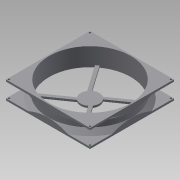
# Autodesk Inventor part: fan_body
Saved by Autodesk Inventor 2015 (Build 190159000, 159)
## iProperties
Created: 2015-05-21
Part Number: fan_body
Material: Generic
Document SubType Name: Modeling
Designer: Joe Sheldon
Density: 1 g/cm^3
Appearance: Default
Author: Joe Sheldon
Autodesk Inventor part; units mm, degrees
ref_plane "YZ Plane" through (0, 0, 0) normal (1, 0, 0) x (0, 1, 0)
ref_plane "XZ Plane" through (0, 0, 0) normal (0, 1, 0) x (-1, 0, 0)
ref_plane "XY Plane" through (0, 0, 0) normal (0, 0, 1) x (1, 0, 0)
sketch "Sketch1" plane through (0, 0, 0) normal (0, 1, 0) x (-1, 0, 0)
  line L0 (0, 0) -> (88.9, 0)
  line L1 (88.9, 0) -> (88.9, -88.9)
  line L2 (88.9, -88.9) -> (0, -88.9)
  line L3 (0, -88.9) -> (0, 0)
  circle A0 centre (44.45, -44.45) radius 43.18
  dimension "d0" = 88.9
  dimension "d1" = 88.9
  dimension "d2" = 86.36
  constraints: 8 end point, 2 parallel, 1 centre point, 1 horizontal, 1 perpendicular
  measures "d0" distance of L1.end L2.end
  measures "d1" distance of L0.end L1.end
  measures "d2" diameter of A0
extrude "Extrusion1" add sketch "Sketch1" along normal blind 23.114
sketch "Sketch2" plane through (0, 23.114, 0) normal (0, 1, 0) x (1, 0, 0)
  line L0 (0, 0) -> (-1.6002, 0)
  line L1 (-1.6002, 0) -> (-1.6002, 1.6002)
  line L2 (-1.6002, 1.6002) -> (0, 1.6002)
  line L3 (0, 1.6002) -> (0, 0)
  line L4 (-88.9, 0) -> (-87.2998, 0)
  line L5 (-87.2998, 0) -> (-87.2998, 1.6002)
  line L6 (-87.2998, 1.6002) -> (-88.9, 1.6002)
  line L7 (-88.9, 1.6002) -> (-88.9, 0)
  line L8 (-88.9, 88.9) -> (-87.2998, 88.9)
  line L9 (-87.2998, 88.9) -> (-87.2998, 87.2998)
  line L10 (-87.2998, 87.2998) -> (-88.9, 87.2998)
  line L11 (-88.9, 87.2998) -> (-88.9, 88.9)
  line L12 (0, 88.9) -> (-1.6002, 88.9)
  line L13 (-1.6002, 88.9) -> (-1.6002, 87.2998)
  line L14 (-1.6002, 87.2998) -> (0, 87.2998)
  line L15 (0, 87.2998) -> (0, 88.9)
  circle A0 centre (-87.2998, 1.6002) radius 0.9525
  circle A1 centre (-87.2998, 87.2998) radius 0.9525
  circle A2 centre (-1.6002, 87.2998) radius 0.9525
  circle A3 centre (-1.6002, 1.6002) radius 0.9525
  dimension "d5" = 1.6002
  dimension "d6" = 1.6002
  dimension "d7" = 1.6002
  dimension "d8" = 1.6002
  dimension "d9" = 1.6002
  dimension "d10" = 1.6002
  dimension "d11" = 1.6002
  dimension "d12" = 1.6002
  dimension "d13" = 1.905
  dimension "d14" = 1.905
  dimension "d15" = 1.905
  dimension "d16" = 1.905
  constraints: 32 end point, 8 parallel, 4 centre point, 4 coincident, 4 horizontal, 4 perpendicular
  measures "d5" distance of L1.end L2.end
  measures "d6" distance of L0.end L1.end
  measures "d7" distance of L6.end L5.end
  measures "d8" distance of L5.end L4.end
  measures "d9" distance of L9.end L10.end
  measures "d10" distance of L8.end L9.end
  measures "d11" distance of L14.end L13.end
  measures "d12" distance of L13.end L12.end
  measures "d13" diameter of A0
  measures "d14" diameter of A1
  measures "d15" diameter of A2
  measures "d16" diameter of A3
extrude "Extrusion2" cut sketch "Sketch2" against normal blind 29.464 contours A3 L2 L1 | L1 L2 A3 | A0 L6 L5 | L5 L6 A0 | A1 L10 L9 | L9 L10 A1 | A2 L14 L13 | L13 L14 A2
sketch "Sketch3" plane through (-88.9, 0, 0) normal (0, 0, 1) x (1, 0, 0)
  line L0 (88.9, 0) -> (0, 0) projected
  line L1 (88.9, 0) -> (88.9, 23.114) projected
  line L2 (0, 23.114) -> (88.9, 23.114) projected
  line L3 (0, 0) -> (0, 23.114) projected
  line L4 (88.9, 0) -> (88.9, 23.114) projected
  line L5 (0, 23.114) -> (88.9, 23.114)
  line L6 (88.9, 23.114) -> (88.9, 21.082)
  line L7 (88.9, 21.082) -> (0, 21.082)
  line L8 (0, 21.082) -> (0, 23.114)
  dimension "d19" = 2.032
  constraints: 8 end point, 2 parallel, 1 horizontal, 1 perpendicular, 1 point on line
  measures "d19" distance of L5.end L6.end
extrude "Extrusion3" cut sketch "Sketch3" against normal blind 96.139 contours L0 L3 L7 L1
sketch "Sketch4" plane through (0, 23.114, 0) normal (0, 1, 0) x (1, 0, 0)
  circle A0 centre (-1.6002, 1.6002) radius 0.9525 projected
  circle A1 centre (-87.2998, 87.2998) radius 0.9525 projected
  circle A2 centre (-87.2998, 1.6002) radius 0.9525 projected
  circle A3 centre (-1.6002, 87.2998) radius 0.9525 projected
  circle A4 centre (-44.45, 44.45) radius 43.18 projected
  line L0 (-88.9, 0) -> (0, 0) projected
  line L1 (0, 0) -> (0, 88.9) projected
  line L2 (0, 88.9) -> (-88.9, 88.9) projected
  line L3 (-88.9, 88.9) -> (-88.9, 0) projected
  circle A5 centre (-44.45, 44.45) radius 44.348
  constraints: 1 centre point
extrude "Extrusion4" add sketch "Sketch4" along normal blind 7.62 contours A5
chamfer "Chamfer1" distance 4.7625 angle 45 1 edges at (-88.798, 23.114, -44.45)
mirror "Mirror1" about plane through (-44.45, 30.734, -44.45) normal (0, 1, 0) of "Extrusion1", "Extrusion4", "Chamfer1", "Extrusion2"
sketch "Sketch5" plane through (-88.9, 61.468, 0) normal (0, 0, 1) x (1, 0, 0)
  line L0 (88.9, 0) -> (0, 0) projected
  line L1 (0, 0) -> (0, -23.114) projected
  line L2 (0, -23.114) -> (23.5685, -23.114) projected
  line L3 (65.3315, -23.114) -> (88.9, -23.114) projected
  line L4 (88.9, 0) -> (88.9, -23.114) projected
  line L5 (88.9, 0) -> (88.9, -23.114) projected
  line L6 (0, -23.114) -> (88.9, -23.114)
  line L7 (88.9, -23.114) -> (88.9, -21.082)
  line L8 (88.9, -21.082) -> (0, -21.082)
  line L9 (0, -21.082) -> (0, -23.114)
  point P0 (88.9, -61.468)
  dimension "d27" = 2.032
  constraints: 8 end point, 2 parallel, 1 horizontal, 1 horizontal alignment, 1 perpendicular, 1 point on line
  measures "d27" distance of L7.end L6.end
extrude "Extrusion5" cut sketch "Sketch5" against normal blind 106.045 contours L4 L8 L1 L0
sketch "Sketch7" plane through (-88.9, 21.082, 0) normal (0, -1, 0) x (1, 0, 0)
  line L0 (75.9799, 0) -> (78.7808, -1.9598)
  line L1 (78.7808, -1.9598) -> (49.7901, -43.3923)
  line L2 (49.7901, -43.3923) -> (46.9892, -41.4325)
  line L3 (46.9892, -41.4325) -> (75.9799, 0)
  point P0 (88.9, 0)
  constraints: 8 end point, 2 parallel, 1 perpendicular
extrude "Extrusion6" add sketch "Sketch7" against normal blind 2.032
pattern_circular "Circular Pattern1" count 4 over 360 about axis through (-44.45, 61.468, -44.45) along (0, 1, 0) of "Extrusion6"
sketch "Sketch8" plane through (-88.9, 21.082, 0) normal (0, -1, 0) x (1, 0, 0)
  arc A0 (23.5685, 0) -> (0, -23.5685) centre (44.45, -44.45) ccw projected
  circle A1 centre (44.45, -44.45) radius 44.348 projected
  circle A2 centre (44.45, -44.45) radius 9.8431
  point P0 (88.9, 0)
  constraints: 1 centre point, 1 coincident
extrude "Extrusion7" add sketch "Sketch8" against normal blind 2.032 contours A2
sketch "Sketch9" plane through (-88.9, 23.114, 0) normal (0, 1, 0) x (1, 0, 0)
  point P0 (88.9, 0)
body "Solid1"
